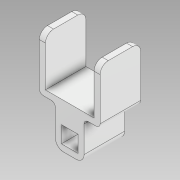
# Autodesk Inventor part: fuselage_tail_interface_airfoiled
Saved by Autodesk Inventor 2021 (Build 250183000, 183)
## iProperties
Created: 2020-11-20
Part Number: fuselage_tail_interface_airfoiled
Material: ABS Plastic
Document SubType Name: Modeling
Designer: Paco
Density: 1.06 g/cm^3
Appearance: Smooth - White
Mass: 1.13699 g
Surface Area: 13.342 cm^2
Volume: 1.07263 cm^3
Author: Paco
Autodesk Inventor part; units mm, degrees
ref_plane "YZ Plane" through (0, 0, 0) normal (1, 0, 0) x (0, 1, 0)
ref_plane "XZ Plane" through (0, 0, 0) normal (0, 1, 0) x (-1, 0, 0)
ref_plane "XY Plane" through (0, 0, 0) normal (0, 0, 1) x (1, 0, 0)
sketch "Sketch1" plane through (0, 0, 0) normal (0, 0, 1) x (1, 0, 0)
  line L0 (-2.05, 2.05) -> (2.05, 2.05)
  line L1 (2.05, 2.05) -> (2.05, -2.05)
  line L2 (2.05, -2.05) -> (-2.05, -2.05)
  line L3 (-2.05, -2.05) -> (-2.05, 2.05)
  line L4 (0, 2.05) -> (0, -2.05) construction
  line L5 (0, 7.5) -> (-15.55, 7.5)
  line L6 (-15.55, 7.5) -> (-15.55, 6)
  line L7 (-15.55, 6) -> (-3.55, 6)
  line L8 (-3.55, 6) -> (-3.55, -6)
  line L9 (-3.55, -6) -> (-15.55, -6)
  line L10 (-15.55, -6) -> (-15.55, -7.5)
  line L11 (-15.55, -7.5) -> (-0.55, -7.5)
  line L12 (-2.05, 0) -> (2.05, 0) construction
  line L13 (0, 7.5) -> (15.55, 7.5)
  line L14 (15.55, 7.5) -> (15.55, 6)
  line L15 (15.55, 6) -> (3.55, 6)
  line L16 (3.55, 6) -> (3.55, -6)
  line L17 (3.55, -6) -> (15.55, -6)
  line L18 (15.55, -6) -> (15.55, -7.5)
  line L19 (15.55, -7.5) -> (-0.55, -7.5)
  line L20 (-2.05, 2.05) -> (2.05, -2.05) construction
  line L21 (2.05, 2.05) -> (-2.05, -2.05) construction
  line L22 (0, 7.5) -> (0, 2.05) construction
  line L23 (-3.55, 6) -> (-3.55, 7.5)
  line L24 (-3.55, -6) -> (-3.55, -7.5)
  line L25 (3.55, 6) -> (3.55, 7.5)
  line L26 (3.55, -6) -> (3.55, -7.5)
  point P0 (0, 0)
  point P1 (0, 0)
  point P2 (0, 0)
  dimension "d3" = 4.1
  dimension "d4" = 4.1
  dimension "d5" = 12
  dimension "d6" = 1.5
  dimension "d7" = 1.5
  dimension "d8" = 5.45
  dimension "d9" = 5.45
  dimension "d10" = 1.5
  dimension "d11" = 12
  dimension "d37" = 15
  constraints: 54 end point, 10 point on line, 8 perpendicular, 6 midpoint, 6 symmetric about line, 2 horizontal, 2 parallel, 1 coincident, 1 vertical, 1 other
  measures "d3" distance of L0.start L0.end
  measures "d4" distance of L0.end L1.end
  measures "d5" distance between parallel lines of L9 L7
  measures "d6" distance of L5.end L6.end
  measures "d7" distance of L9.end L10.end
  measures "d8" distance between parallel lines of L0 L5
  measures "d9" distance between parallel lines of L11 L2
  measures "d10" distance between parallel lines of L8 L3
  measures "d11" distance of L6.end L7.end
  measures "d37" distance between parallel lines of L11 L5
extrude "Extrusion1" add sketch "Sketch1" along normal blind 10 contours L13 L25 L16 L26 L19 L11 L24 L8 L23 L5
sketch "Sketch5" plane through (0, 0, 10) normal (0, 0, 1) x (1, 0, 0)
  line L0 (6, 19.5) -> (7.5, 19.5)
  line L1 (7.5, 19.5) -> (7.5, 7.5)
  line L2 (7.5, 7.5) -> (6, 7.5)
  line L3 (6, 7.5) -> (6, 19.5)
  line L4 (3.55, 7.5) -> (-3.55, 7.5) projected
  line L5 (3.55, -7.5) -> (3.55, 7.5) projected
  line L6 (0, 0) -> (0, 23.4065) construction
  point P0 (15.55, 7.5)
  point P1 (-15.55, 7.5)
  point P2 (3.55, -6)
  point P3 (3.55, 6)
  dimension "d41" = 1.5
  dimension "d42" = 12
  dimension "d47" = 6
  constraints: 10 end point, 2 parallel, 2 vertical, 1 collinear, 1 horizontal, 1 perpendicular
  measures "d41" distance of L0.start L0.end
  measures "d42" distance of L0.end L1.end
  measures "d47" distance between parallel lines of L3 L6
extrude "Extrusion5" add sketch "Sketch5" against normal up to surface (10 mm away)
mirror "Mirror1" about plane through (0, 0, 0) normal (1, 0, 0) of "Extrusion5"
sketch "Sketch7" plane through (0, 0, 10) normal (0, 0, 1) x (1, 0, 0)
  line L0 (-7.5, 19.5) -> (-7.5, 7.5) projected
  line L1 (-7.5, 7.5) -> (7.5, 7.5)
  line L2 (7.5, 7.5) -> (7.5, 6)
  line L3 (7.5, 6) -> (-7.5, 6)
  line L4 (-7.5, 6) -> (-7.5, 7.5)
  line L5 (7.5, 7.5) -> (7.5, 19.5) projected
  point P0 (0, 0)
  dimension "d53" = 1.5
  constraints: 8 end point, 2 parallel, 1 collinear, 1 horizontal, 1 perpendicular
  measures "d53" distance between parallel lines of L1 L3
extrude "Extrusion7" add sketch "Sketch7" against normal up to surface (10 mm away)
fillet "Fillet3" radius 1 4 edges at (-3.55, 6, 5) (3.55, 6, 5) (7.5, 6, 5) (-7.5, 6, 5)
sketch "Sketch8" plane through (0, 0, 10) normal (0, 0, 1) x (1, 0, 0)
  line L0 (-3.55, -3.55) -> (3.55, -3.55)
  line L1 (3.55, -3.55) -> (3.55, -7.5)
  line L2 (3.55, -7.5) -> (-3.55, -7.5)
  line L3 (-3.55, -7.5) -> (-3.55, -3.55)
  line L4 (2.05, -2.05) -> (-2.05, -2.05) projected
  line L5 (3.55, -7.5) -> (3.55, 5) projected
  line L6 (-3.55, 5) -> (-3.55, -7.5) projected
  line L7 (-3.55, -7.5) -> (3.55, -7.5) projected
  point P0 (0, 0)
  dimension "d57" = 1.5
  constraints: 8 end point, 3 collinear, 2 parallel, 1 horizontal, 1 perpendicular
  measures "d57" distance between parallel lines of L0 L4
extrude "Extrusion8" cut sketch "Sketch8" against normal blind 10
fillet "Fillet4" radius 2 4 edges at (-6.75, 19.5, 10) (-6.75, 19.5, 0) (6.75, 19.5, 0) (6.75, 19.5, 10)
fillet "Fillet5" radius 2 2 edges at (3.55, -3.55, 5) (-3.55, -3.55, 5)
equation "\"d7\" = d6"
equation "\"d8\" = d9"
body "Solid1"
